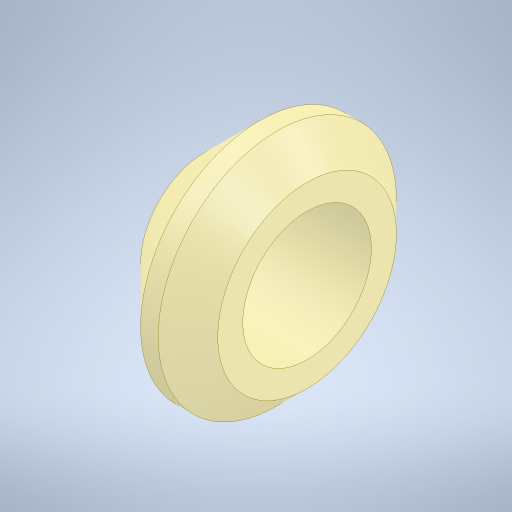
# Autodesk Inventor part: Spacer
Saved by Autodesk Inventor 2023.2 (Build 272271000, 271)
## iProperties
Created: 2023-04-29
Part Number: Spacer
Material: Nylon 6/6
Document SubType Name: Modeling
Designer: Nathan Cai
Density: 1.13 g/cm^3
Appearance: Nylon 6
Author: Nathan Cai
Autodesk Inventor part; units mm, degrees
ref_plane "YZ Plane" through (0, 0, 0) normal (1, 0, 0) x (0, 1, 0)
ref_plane "XZ Plane" through (0, 0, 0) normal (0, 1, 0) x (-1, 0, 0)
ref_plane "XY Plane" through (0, 0, 0) normal (0, 0, 1) x (1, 0, 0)
sketch "Sketch1" plane through (0, 0, 0) normal (0, 1, 0) x (-1, 0, 0)
  line L0 (0, 0) -> (5.4483, 0)
  line L1 (5.4483, 0) -> (5.4483, -3.429) construction
  line L2 (5.4483, -3.429) -> (0, -3.429)
  line L3 (0, -3.429) -> (0, 0) construction
  line L4 (5.4483, -3.429) -> (0, -3.429)
  line L5 (0, -3.429) -> (0, -6.35)
  line L6 (0, -6.35) -> (5.4483, -6.35)
  line L7 (5.4483, -6.35) -> (5.4483, -3.429)
  dimension "d0" = 5.4483
  dimension "d1" = 3.429
  dimension "d2" = 6.35
  constraints: 16 end point, 4 parallel, 2 horizontal, 2 perpendicular, 1 point on line
  measures "d0" distance of L1.end L2.end
  measures "d1" distance between parallel lines of L0 L2
  measures "d2" distance between parallel lines of L0 L6
revolve "Revolution1" add sketch "Sketch1" angle 360 about axis through (0, 0, 0) along (-1, 0, 0)
chamfer "Chamfer1" distance 2.921 angle 45 1 edges at (-5.4483, 0, 6.35)
chamfer "Chamfer2" distance 1.5875 angle 45 1 edges at (0, 0, 6.35)
body "Solid1"
